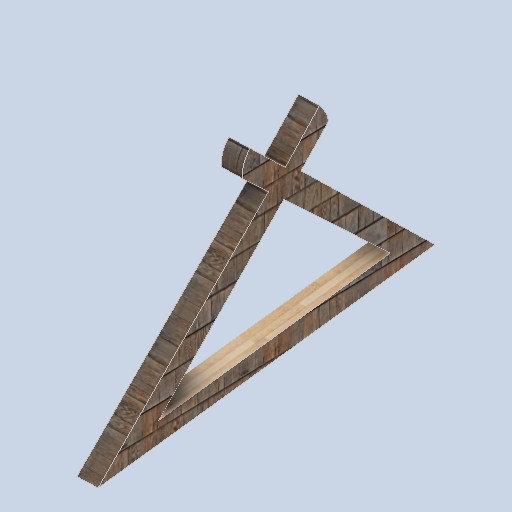
# Autodesk Inventor part: panel_block_02
Saved by Autodesk Inventor 2024.2 (Build 282272000, 272)
## iProperties
Created: 2024-05-21
Part Number: panel_block_02
Material: Wood (Maple)
Document SubType Name: Modeling
Designer: LOSTER_1
Density: 0.67 g/cm^3
Appearance: Natural Maple - Glossy Dark Tint
Author: LOSTER_1
Autodesk Inventor part; units mm, degrees
sketch "Sketch1" plane through (0, 0, 0) normal (0, 0, 1) x (1, 0, 0)
  line L0 (2948.6488, 634.5525) -> (2841.4489, 559.4904)
  line L1 (2841.4489, 559.4904) -> (2956.2003, 395.6085)
  line L2 (2956.2003, 395.6085) -> (3063.4001, 470.6706)
  line L3 (1051.1773, 2444.1167) -> (976.8907, 2338.0244)
  line L4 (976.8907, 2338.0244) -> (1140.7211, 2223.3091)
  line L5 (1140.7211, 2223.3091) -> (1215.0077, 2329.4014)
  line L6 (-383.8501, 3232.1868) -> (-383.8501, 3052.6308)
  arc A0 (4065.9398, -2152.4924) -> (-383.8501, 3052.6308) centre (-4485.4868, -4958.3977) ccw
  arc A1 (1051.1773, 2444.1167) -> (-383.8501, 3232.1868) centre (-3980.604, -5017.8654) ccw
  arc A2 (2948.6488, 634.5525) -> (1215.0077, 2329.4014) centre (-4152.392, -4894.9339) ccw
  arc A3 (4300.883, -1939.8955) -> (3063.4001, 470.6706) centre (-4233.2291, -4798.0297) ccw
  arc A4 (4065.9398, -2152.4924) -> (4300.883, -1939.8955) centre (3657.2708, -1464.7499) ccw
  point P0 (0, 0)
  point P1 (4065.924, -2152.4924)
  point P2 (4065.924, -2152.4924)
  dimension "d8" = 9000
  dimension "d9" = 9000
  dimension "d10" = 9000
  dimension "d11" = 9000
  dimension "d12" = 800
  constraints: 14 end point, 10 point on circle, 5 centre point, 4 perpendicular, 1 coincident, 1 vertical
  measures "d8" radius of A0
  measures "d9" radius of A1
  measures "d10" radius of A2
  measures "d11" radius of A3
  measures "d12" radius of A4
ref_plane "Work Plane2" through (0, 0, -7900) normal (0, 0, 1) x (1, 0, 0)
ref_plane "Work Plane1" through (0, 0, 0) normal (0, 0, 1) x (1, 0, 0)
sketch "Sketch2" plane through (0, 0, -7900) normal (0, 0, 1) x (1, 0, 0)
  arc A0 (895.257, 3171.2695) -> (-383.8658, 4018.7524) centre (-4697.1096, -3880.3569) ccw projected
  line L0 (-383.8658, 4018.7524) -> (-383.8658, 3839.1061) projected
  arc A1 (4065.924, -2152.4924) -> (-383.8658, 3839.1061) centre (-4733.9746, -4039.7614) ccw projected
  line L1 (895.257, 3171.2695) -> (830.4728, 3059.0601) projected
  line L2 (830.4728, 3059.0601) -> (1003.6891, 2959.0536) projected
  line L3 (1068.4733, 3071.2631) -> (1003.6891, 2959.0536) projected
  arc A2 (2750.1419, 1279.62) -> (1068.4733, 3071.2631) centre (-4591.4319, -3926.2703) ccw projected
  line L4 (2750.1419, 1279.62) -> (2643.8882, 1205.2246) projected
  line L5 (2643.8882, 1205.2246) -> (2759.146, 1041.7698) projected
  line L6 (2865.5448, 1116.2711) -> (2759.146, 1041.7698) projected
  arc A3 (4310.9102, -1926.005) -> (2865.5448, 1116.2711) centre (-4397.3898, -4198.7812) ccw projected
  arc A4 (4065.924, -2152.4924) -> (4310.9102, -1926.005) centre (3657.2831, -1464.7333) ccw
  point P0 (0, 0)
  dimension "d7" = 800
  constraints: 2 point on circle, 1 centre point
  measures "d7" radius of A4
loft "Loft1" add profiles "Sketch1", "Sketch2"
ref_plane "Work Plane3" through (2500, 0, 0) normal (1, 0, 0) x (0, 1, 0)
sketch "Sketch3" plane through (2500, 0, 0) normal (1, 0, 0) x (0, 1, 0)
  line L0 (2569.5835, -3718.0946) -> (1551.2045, -2616.5476)
  line L1 (1551.2045, -2616.5476) -> (1738.7871, -4630.7013)
  line L2 (1738.7871, -4630.7013) -> (2569.5835, -3718.0946)
  line L3 (4228.9662, 279.606) -> (-2269.9695, 279.606)
  line L4 (-2269.9695, 279.606) -> (-2269.9695, -8192.2559)
  line L5 (-2269.9695, -8192.2559) -> (4228.9662, -8192.2559)
  line L6 (4228.9662, -8192.2559) -> (4228.9662, 279.606)
  point P0 (0, 0)
  constraints: 14 end point, 2 parallel, 1 horizontal, 1 perpendicular
extrude "Extrusion1" cut sketch "Sketch3" along normal through all both and the other way through all
ref_plane "Work Plane4" through (1945.737, 1551.2045, -2616.5476) normal (0, -0.9956912, -0.0927309) x (1, 0, 0)
sketch "Sketch5" plane through (1945.737, 1551.2045, -2616.5476) normal (0, -0.9956912, -0.0927309) x (1, 0, 0)
  line L0 (347.8734, 0) -> (290.3896, -2022.8698)
  point P0 (-1945.737, 2749.1181)
  constraints: 2 end point
ref_plane "Work Plane5" through (2293.6104, 1551.2045, -2616.5476) normal (-0.6425282, -0.7644369, -0.052856) x (-0.0284055, 0.0926935, -0.9952894)
sketch "Sketch6" plane through (2293.6104, 1551.2045, -2616.5476) normal (-0.6425282, -0.7644369, -0.052856) x (-0.0284055, 0.0926935, -0.9952894)
  line L0 (-1061.9028, -2252.9112) -> (2197.0944, -2252.9112)
  line L1 (2197.0944, -2252.9112) -> (2197.0944, 343.7273)
  line L2 (2197.0944, 343.7273) -> (-1061.9028, 343.7273)
  line L3 (-1061.9028, 343.7273) -> (-1061.9028, -2252.9112)
  point P0 (-2682.8576, -979.2829)
  constraints: 8 end point, 2 parallel, 1 horizontal, 1 perpendicular
extrude "Extrusion2" cut sketch "Sketch6" against normal through all
ref_plane "Work Plane6" through (2293.6104, 1551.2045, -2616.5476) normal (-0.9995965, -0.0026341, 0.0282831) x (-0.0284055, 0.0926935, -0.9952894)
sketch "Sketch7" plane through (2293.6104, 1551.2045, -2616.5476) normal (-0.6425282, -0.7644369, -0.052856) x (-0.0284055, 0.0926935, -0.9952894)
  line L0 (0, 0) -> (1222.5973, -1418.5767) projected
  line L1 (1222.5973, -1418.5767) -> (2023.6864, 0) projected
  point P0 (-2682.8576, -979.2829)
  constraints: 1 horizontal alignment
sketch "Sketch8" plane through (2293.6104, 1551.2045, -2616.5476) normal (-0.9995965, -0.0026341, 0.0282831) x (-0.0284055, 0.0926935, -0.9952894)
  line L0 (0, 0) -> (1222.5973, -911.8435) projected
  spline S0 degree 4 poles (2023.6864, 0) (1891.4174, -0.0605) (1759.1485, -0.1112) (1626.8795, -0.1518) (1361.543, -0.2126) (1228.4756, -0.2325) (1095.4081, -0.2417) (831.8573, -0.2379) (701.374, -0.2253) (570.8907, -0.2017) (330.3055, -0.1374) (220.2037, -0.0999) (110.1018, -0.0542) (0, 0) knots 0 0 0 0 0 0.261442 0.261442 0.261442 0.524462 0.524462 0.524462 0.782374 0.782374 0.782374 1 1 1 1 1 projected
  line L1 (1222.5973, -911.8435) -> (2023.6864, 0) projected
  point P0 (-2682.8576, 1301.8858)
  constraints: 1 horizontal alignment
loft "Loft2" add profiles "Sketch8" section 1 edges at (1733.119, 2060.394, -3167.3211) (2264.5827, 1645.2339, -3623.5941) (1704.3771, 2154.1853, -4174.3979)
sketch "Sketch9" plane through (2293.6104, 1551.2045, -2616.5476) normal (-0.9995965, -0.0026341, 0.0282831) x (-0.0284055, 0.0926935, -0.9952894)
  line L0 (1222.5973, -911.8435) -> (0, 0) projected
  line L1 (2023.6864, 0) -> (1222.5973, -911.8435) projected
  spline S0 degree 4 poles (0, 0) (110.1018, -0.0542) (220.2037, -0.0999) (330.3055, -0.1374) (570.8907, -0.2017) (701.374, -0.2253) (831.8573, -0.2379) (1095.4081, -0.2417) (1228.4756, -0.2325) (1361.543, -0.2126) (1626.8795, -0.1518) (1759.1485, -0.1112) (1891.4174, -0.0605) (2023.6864, 0) knots 0 0 0 0 0 0.217626 0.217626 0.217626 0.475538 0.475538 0.475538 0.738558 0.738558 0.738558 1 1 1 1 1 projected
  point P0 (-2682.8576, 1301.8858)
  constraints: 1 horizontal alignment
extrude "Extrusion3" add sketch "Sketch9" against normal blind 1
sketch "Sketch10" plane through (2294.61, 1551.2071, -2616.5759) normal (0.9995965, 0.0026341, -0.0282831) x (-0.0284055, 0.0926935, -0.9952894)
  line L0 (2023.6864, 0) -> (1222.5973, 911.8435) projected
  line L1 (1222.5973, 911.8435) -> (0, 0) projected
  point P0 (-2682.8576, -1301.8858)
  constraints: 1 horizontal alignment
sketch "Sketch11" plane through (2294.61, 1551.2071, -2616.5759) normal (0.9995965, 0.0026341, -0.0282831) x (-0.0284055, 0.0926935, -0.9952894)
  line L0 (-1104.2744, 1764.8294) -> (3009.0866, 1764.8294)
  line L1 (3009.0866, 1764.8294) -> (3009.0866, -1120.984)
  line L2 (3009.0866, -1120.984) -> (-1104.2744, -1120.984)
  line L3 (-1104.2744, -1120.984) -> (-1104.2744, 1764.8294)
  point P0 (-2682.8576, -1301.8858)
  constraints: 8 end point, 2 parallel, 1 horizontal, 1 perpendicular
extrude "Extrusion4" cut sketch "Sketch11" against normal through all
ref_plane "Work Plane7" through (2259.8815, 2572.4485, -3748.8579) normal (-0.9995965, -0.0026341, 0.0282831) x (0.02277, -0.6695833, 0.7423878)
sketch "Sketch12" plane through (2259.8815, 2572.4485, -3748.8579) normal (-0.9995965, -0.0026341, 0.0282831) x (0.02277, -0.6695833, 0.7423878)
  line L0 (1824.1754, 71.0087) -> (-191.8191, -1432.5702)
  line L1 (-191.8191, -1432.5702) -> (-218.3749, -1452.3762)
  line L2 (1355.6088, -93.5273) -> (-48.5024, -1138.6261)
  line L3 (-48.5024, -1138.6261) -> (43.4592, -46.5069)
  line L4 (-218.3749, -1452.3762) -> (-129.6551, -49.5311)
  line L5 (1824.1754, 71.0087) -> (56.688, 110.5959)
  line L6 (56.688, 110.5959) -> (79.2582, 378.6347)
  line L7 (-129.6551, -49.5311) -> (-422.1869, -34.2052)
  line L8 (-97.0049, 90.8023) -> (-72.3771, 459.6792)
  line L9 (-97.0049, 90.8023) -> (-461.7897, 110.5959)
  arc A0 (-461.7897, 110.5959) -> (-422.1869, -34.2052) centre (-203.8576, 103.3236) ccw
  arc A1 (79.2582, 378.6347) -> (-72.3771, 459.6792) centre (-80.6938, 261.7407) ccw
  line L10 (43.4592, -46.5069) -> (1355.6088, -93.5273)
  point P0 (4454.1178, 560.366)
  point P1 (0, 0)
  point P2 (1525.1894, 0)
  point P3 (-97.0049, -1209.8729)
  point P4 (1451.8368, -21.9036)
  constraints: 22 end point, 4 point on circle, 2 centre point
extrude "Extrusion5" add sketch "Sketch12" against normal blind 150
ref_plane "Work Plane8" through (2334.8512, 2572.6461, -3750.9792) normal (-0.9995965, -0.0026341, 0.0282831) x (0.02277, -0.6695833, 0.7423878)
sketch "Sketch14" plane through (2334.8512, 2572.6461, -3750.9792) normal (-0.9995965, -0.0026341, 0.0282831) x (0.02277, -0.6695833, 0.7423878)
  line L0 (1451.8368, -21.9036) -> (43.4592, -46.5069) projected
  line L1 (43.4592, -46.5069) -> (-48.5024, -1138.6261) projected
  line L2 (-48.5024, -1138.6261) -> (1355.6088, -93.5273) projected
  line L3 (-48.5024, -1138.6261) -> (43.4592, -46.5069) projected
  line L4 (36.357, -130.8518) -> (1354.1445, -94.6172)
  line L5 (29.9819, -206.5611) -> (1254.1697, -169.0298)
  line L6 (23.4479, -284.1574) -> (1145.7195, -249.7507)
  line L7 (16.9375, -361.4743) -> (1037.66, -330.1809)
  line L8 (11.2021, -429.586) -> (925.5677, -413.6127)
  line L9 (5.2661, -500.0812) -> (833.993, -481.773)
  line L10 (5.2661, -580.2648) -> (718.4048, -567.8068)
  line L11 (5.2661, -580.2648) -> (-1.4957, -580.383)
  line L12 (-7.9772, -657.3559) -> (615.2506, -644.5859)
  line L13 (-14.4897, -734.6974) -> (512.2276, -721.2673)
  line L14 (-20.8834, -810.6278) -> (426.4206, -798.3271)
  line L15 (-26.6611, -879.2427) -> (308.1889, -873.136)
  line L16 (-32.3399, -946.6834) -> (221.1278, -937.9367)
  line L17 (-37.3457, -1006.1304) -> (133.6992, -1003.011)
  line L18 (-41.9227, -1060.4869) -> (56.4792, -1060.4869)
  line L19 (1355.6088, -93.5273) -> (-48.5024, -1138.6261) projected
  line L20 (116.3671, -52.6461) -> (14.2049, -1091.9522)
  line L21 (190.5781, -52.6461) -> (82.9233, -1040.8042)
  line L22 (190.5781, -52.6461) -> (191.5287, -43.9202)
  line L23 (116.3671, -52.6461) -> (117.0971, -45.2205)
  line L24 (264.8096, -42.6401) -> (168.5004, -977.108)
  line L25 (335.0568, -41.4129) -> (244.4471, -920.5799)
  line L26 (405.5718, -40.181) -> (320.6833, -863.8362)
  line L27 (43.4592, -46.5069) -> (1451.8368, -21.9036) projected
  line L28 (494.8216, -38.6219) -> (401.4074, -815.2786)
  line L29 (584.5837, -37.0538) -> (494.8216, -734.2227)
  line L30 (673.0821, -35.5078) -> (584.5837, -667.4116)
  line L31 (761.0304, -33.9714) -> (682.5265, -594.5115)
  line L32 (845.2654, -32.4999) -> (776.3341, -524.6893)
  line L33 (922.1945, -31.156) -> (862.0055, -460.9229)
  line L34 (1000.074, -29.7955) -> (948.7353, -396.3688)
  line L35 (1079.0786, -28.4154) -> (1030.8888, -335.2208)
  line L36 (1150.7176, -27.1639) -> (1111.7893, -275.0055)
  line L37 (1222.0396, -25.918) -> (1192.3317, -215.0567)
  line L38 (1300.3477, -24.55) -> (1272.1344, -155.6584)
  line L39 (1372.2211, -23.2944) -> (1361.9285, -88.8235)
  point P0 (4454.1178, 560.366)
  point P1 (108.8756, -128.8578)
  point P2 (182.4957, -126.8335)
  point P3 (174.2918, -202.1368)
  point P4 (101.4529, -204.3699)
  point P5 (79.4317, -428.3941)
  point P6 (149.7761, -427.1652)
  point P7 (142.1618, -497.0569)
  point P8 (72.531, -498.5951)
  point P9 (49.4829, -733.0662)
  point P10 (116.6363, -731.354)
  point P11 (108.3871, -807.0729)
  point P12 (42.0287, -808.8978)
  point P13 (256.3417, -124.803)
  point P14 (326.6617, -122.8694)
  point P15 (318.9492, -197.7019)
  point P16 (248.6062, -199.8585)
  point P17 (240.6042, -277.4998)
  point P18 (310.9472, -275.3432)
  point P19 (302.9741, -352.7049)
  point P20 (232.6311, -354.8615)
  point P21 (225.3153, -425.8456)
  point P22 (295.5625, -424.6184)
  point P23 (288.4297, -493.8255)
  point P24 (218.149, -495.3782)
  point P25 (209.7685, -576.6923)
  point P26 (280.0157, -575.4652)
  point P27 (272.1674, -651.6157)
  point P28 (201.8983, -653.0555)
  point P29 (194.032, -729.3806)
  point P30 (264.3374, -727.5879)
  point P31 (256.5654, -802.9981)
  point P32 (186.2454, -804.9319)
  point P33 (750.2112, -111.2233)
  point P34 (834.565, -108.9039)
  point P35 (824.2986, -182.2089)
  point P36 (739.9073, -184.7961)
  point P37 (729.0212, -262.5259)
  point P38 (813.4125, -259.9386)
  point P39 (802.5656, -337.3884)
  point P40 (718.1743, -339.9757)
  point P41 (707.3275, -417.4252)
  point P42 (791.5625, -415.9537)
  point P43 (782.1842, -482.9175)
  point P44 (697.8945, -484.7796)
  point P45 (911.6025, -106.7856)
  point P46 (989.5918, -104.6412)
  point P47 (979.3944, -177.4539)
  point P48 (901.3704, -179.846)
  point P49 (890.4843, -257.5757)
  point P50 (968.5083, -255.1837)
  point P51 (957.6614, -332.6335)
  point P52 (879.6374, -335.0256)
  point P53 (1067.4421, -102.5006)
  point P54 (1139.1944, -100.5276)
  point P55 (1127.8264, -172.9033)
  point P56 (1056.0383, -175.1042)
  point P57 (515.7923, -571.3463)
  point P58 (598.2394, -569.906)
  point P59 (587.7014, -645.1504)
  point P60 (506.0746, -646.8229)
  point P61 (535.2229, -420.4317)
  point P62 (619.3793, -418.9616)
  point P63 (609.8891, -486.7239)
  point P64 (526.4503, -488.5672)
  point P65 (554.8662, -267.8651)
  point P66 (640.9098, -265.2272)
  point P67 (630.0629, -342.677)
  point P68 (544.8979, -345.288)
  point P69 (574.4119, -116.0572)
  point P70 (662.139, -113.645)
  point P71 (651.7959, -187.4975)
  point P72 (564.8706, -190.1624)
  point P73 (350.5307, -574.2333)
  point P74 (430.5679, -572.8351)
  point P75 (421.4603, -648.5567)
  point P76 (342.7044, -650.1704)
  point P77 (366.0774, -423.3866)
  point P78 (448.7168, -421.9429)
  point P79 (440.4749, -490.4665)
  point P80 (358.9784, -492.267)
  point P81 (381.5584, -273.1784)
  point P82 (466.9246, -270.5613)
  point P83 (457.6148, -347.964)
  point P84 (373.5852, -350.5401)
  point P85 (397.2497, -120.9285)
  point P86 (485.2129, -118.5098)
  point P87 (476.268, -192.8788)
  point P88 (389.5603, -195.5371)
  point P89 (35.2249, -878.1141)
  point P90 (100.7778, -876.9186)
  point P91 (93.6509, -942.3357)
  point P92 (28.6916, -944.5773)
  point P93 (64.6049, -579.2282)
  point P94 (133.3405, -578.0275)
  point P95 (124.9949, -654.6313)
  point P96 (57.0561, -656.0234)
  point P97 (93.822, -281.9999)
  point P98 (165.8317, -279.7922)
  point P99 (157.402, -357.1679)
  point P100 (86.2186, -359.3502)
  point P101 (56.4792, -1060.4869)
  point P102 (17.2979, -1060.4869)
  point P103 (22.7488, -1005.0344)
  point P104 (86.9478, -1003.8636)
  point P105 (172.3641, -939.6195)
  point P106 (178.9732, -875.4925)
  point P107 (249.226, -874.2113)
  point P108 (244.4471, -920.5799)
  point P109 (402.9301, -802.6189)
  point P110 (403.37, -798.961)
  point P111 (327.1535, -801.0569)
  point P112 (334.9109, -725.7885)
  point P113 (412.4087, -723.8124)
  point P114 (408.0161, -798.8332)
  point P115 (496.4378, -721.6699)
  point P116 (682.5265, -594.5115)
  point P117 (686.1876, -568.3696)
  point P118 (862.0055, -460.9229)
  point P119 (868.4916, -414.6098)
  point P120 (1030.8888, -335.2208)
  point P121 (1043.8229, -252.8747)
  point P122 (1115.611, -250.6738)
  point P123 (1111.7893, -275.0055)
  point P124 (1199.2969, -170.7121)
  point P125 (1210.6292, -98.5634)
  point P126 (1284.8599, -96.5223)
  point P127 (1272.1344, -155.6584)
  constraints: 68 end point, 12 parallel, 5 point on line, 1 horizontal, 54 other
body "Solid1"
